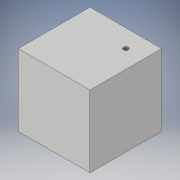
# Autodesk Inventor part: CalibCube
Saved by Autodesk Inventor 2019 (Build 230136000, 136)
## iProperties
Created: 2019-10-07
Part Number: CalibCube
Material: Generic
Document SubType Name: Modeling
Designer: james
Density: 1 g/cm^3
Appearance: Default
Author: james
Autodesk Inventor part; units mm, degrees
ref_plane "YZ Plane" through (0, 0, 0) normal (1, 0, 0) x (0, 1, 0)
ref_plane "XZ Plane" through (0, 0, 0) normal (0, 1, 0) x (-1, 0, 0)
ref_plane "XY Plane" through (0, 0, 0) normal (0, 0, 1) x (1, 0, 0)
sketch "Sketch1" plane through (0, 0, 0) normal (0, 1, 0) x (-1, 0, 0)
  line L0 (19.432, 17.0791) -> (-20.568, 17.0791)
  line L1 (-20.568, 17.0791) -> (-20.568, -22.9209)
  line L2 (-20.568, -22.9209) -> (19.432, -22.9209)
  line L3 (19.432, -22.9209) -> (19.432, 17.0791)
  point P0 (0, 0)
  dimension "d0" = 40
  dimension "d1" = 40
  constraints: 8 end point, 2 parallel, 1 horizontal, 1 perpendicular
  measures "d0" distance of L2.end L0.start
  measures "d1" distance of L0.start L0.end
extrude "Extrusion1" add sketch "Sketch1" along normal blind 40
sketch "Sketch2" plane through (0, 40, 0) normal (0, 1, 0) x (1, 0, 0)
  line L0 (20.568, 22.9209) -> (-19.432, 22.9209) projected
  line L1 (20.568, -17.0791) -> (20.568, 22.9209) projected
  point P0 (0, 0)
  point P1 (10.568, 12.9209)
  dimension "d4" = 10
  dimension "d5" = 10
  measures "d4" distance from line of L0 point (10.568, 12.921)
  measures "d5" distance from line of L1 point (10.568, 12.921)
hole "Hole1" at (10.568, 40, -12.9209) direction (0, -1, 0) diameter 2.6416 depth 10 tip angle 118.188 thread size "6-32 UNC" class "2B" standard "ANSI Unified Screw Threads"
body "Solid1"
